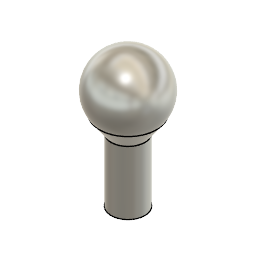
Ball Joint's Baseless Ball (Autodesk Fusion 360 design; units mm, degrees)
Autodesk Fusion 360 part; units mm, degrees
note: some values were not read from the file. Chosen so that the rebuilt part matches the saved one: which bodies a step acts on.
sphere "SpherePrimitive1" add diameter 12 placed x (1, 0, 0) y (0, 1, 0) z (0, 0, 1) at (0, 0, 0) makes body 1
sketch "Sketch2" plane through (0, 0, 0) normal (0, 0, 1) x (1, 0, 0)
  circle A0 centre (0, 0) radius 6
  line L0 (0, 0) -> (3, 0)
  line L1 (2.0741, 19.9496) -> (0, 19.9496)
  line L2 (0, 19.9496) -> (0, 0)
  line L3 (-3, 0) -> (-3, 17.2973)
  line L4 (-2.0741, 19.9496) -> (0, 19.9496)
  line L5 (0, 0) -> (-3, 0)
  line L6 (4.9203, 3.4337) -> (3, 6.1854)
  line L7 (-4.9203, 3.4337) -> (-3, 6.1854)
  line L8 (2.0741, 19.9496) -> (5.0741, 19.9496)
  line L9 (5.0741, 19.9496) -> (9.6681, 19.9496) construction
  line L10 (5.0741, 19.9496) -> (5.0741, 18.7496)
  line L11 (5.0741, 18.7496) -> (3, 17.2973)
  line L12 (-2.0741, 19.9496) -> (-5.0741, 19.9496)
  line L13 (-5.0741, 19.9496) -> (-5.0741, 18.7496)
  line L14 (-5.0741, 18.7496) -> (-3, 17.2973)
  line L15 (3, 0) -> (3, 5.1962)
  line L16 (3, 6.1854) -> (3, 17.2973)
  dimension "d2" = 3
  dimension "d4" = 3
  dimension "d6" = 1.2
  dimension "d7" = 125
  constraint horizontal L0
  constraint vertical L15
  constraint horizontal L1
  constraint vertical L2
  constraint coincident A0.centre L0.start
  constraint symmetric A0.centre L2 L0.start
  constraint symmetric L0.end L2 L3.start
  constraint symmetric L1.start L2 L4.start
  constraint symmetric L1.end L2 L4.end
  constraint coincident L6.end L15
  constraint tangent A0 L6
  constraint coincident A0 L6.start
  constraint symmetric L2 L6.end L7.end
  constraint symmetric L2 L6.start L7.start
  constraint perpendicular L8 L15
  constraint horizontal L9
  constraint perpendicular L9 L10
  constraint symmetric L2 L8.end L12.end
  constraint symmetric L2 L10.end L13.end
  constraint coincident A0 L15.end
  constraint collinear L15 L16
  measures "d2" distance of A0.centre L0.end
  measures "d4" distance of L1.start L8.end
  measures "d6" distance of L8.end L10.end
  measures "d7" angle of L10 L11
revolve "Revolve1" add sketch "Sketch2" angle 360 about axis through (0, 19.9496, 0) along (0, -1, 0) contours A0 L1 L2 L6 L8 L10 L11 L16 bodies 1
copy_body "Body->Comp1" bodies 1 removing the originals makes body 2 in component "ball"
sphere "SpherePrimitive2" add diameter 16 placed x (0, 0, -1) y (0, 1, 0) z (1, 0, 0) at (0, 0, 0) separate body makes body 3
sketch "Sketch4" plane through (0, 0, 0) normal (1, 0, 0) x (0, 0, -1)
  circle A0 centre (0, 0) radius 8
  line L0 (0, 0) -> (3, 0)
  line L1 (3, 0) -> (3, 20)
  line L2 (3, 20) -> (0, 20)
  line L3 (0, 20) -> (0, 0)
  line L4 (3, 20) -> (5, 20)
  line L5 (5, 20) -> (5, 18.5)
  line L6 (5, 18.5) -> (0, 14.999)
  line L7 (6.245, 5) -> (3, 9.053)
  dimension "d10" = 3
  dimension "d11" = 20
  dimension "d12" = 2
  dimension "d13" = 1.5
  dimension "d14" = 125
  dimension "d15" = 15
  constraint horizontal L0
  constraint vertical L1
  constraint horizontal L2
  constraint vertical L3
  constraint coincident A0.centre L0.start
  constraint perpendicular L1 L4
  constraint perpendicular L4 L5
  constraint coincident L3 L6.end
  constraint coincident A0 L7.start
  constraint coincident L1 L7.end
  constraint tangent A0 L7
  measures "d10" distance of A0.centre L0.end
  measures "d11" distance of A0.centre L2.end
  measures "d12" distance of L1.end L4.end
  measures "d13" distance of L4.end L5.end
  measures "d14" angle of L5 L6
  measures "d15" distance of L2 L7.start
revolve "Revolve2" add sketch "Sketch4" angle 360 about axis through (0, 20, 0) along (0, -1, 0) contours A0 L1 L7 | A0 L1 L3 L6 | L1 L2 L3 L6 | L1 L4 L5 L6 bodies 3
sphere "SpherePrimitive3" cut diameter 12 placed x (0, 0, -1) y (0, 1, 0) z (1, 0, 0) at (0, 0, 0) bodies 3
ref_plane "WorkPlane1" through (0, -3, 0) normal (0, 1, 0) x (0, 0, 1)
split "Split1" by plane through (0, -3, 0) normal (0, 1, 0) bodies 3 makes body 4 at (-1.7023, 1.8911, -7.5846)
chamfer "Chamfer1" distance 1 angle 60 1 edges at (-1.879, -3, 4.8445) measured on face at (-1.2767, 1.4183, -5.6884) on bodies 4
sketch "Sketch6" plane through (0, 0, 0) normal (1, 0, 0) x (0, 0, -1)
  line L0 (7.4162, -3) -> (-7.4162, -3) construction
  line L1 (-5, 20) -> (5, 20) construction
  line L2 (-5, 20) -> (-5, 18.5) construction
  line L3 (5, 20) -> (5, 18.5) construction
  line L4 (3, 17.0996) -> (5, 18.5) construction
  line L5 (-3, 17.0996) -> (-5, 18.5) construction
  line L6 (-3, 17.0996) -> (-3, 9.053) construction
  line L7 (3, 17.0996) -> (3, 9.053) construction
  line L8 (-3, 9.053) -> (-6.245, 5) construction
  line L9 (3, 9.053) -> (6.245, 5) construction
  arc A0 (-6.245, 5) -> (-7.4162, -3) centre (0, 0) ccw construction
  arc A1 (7.4162, -3) -> (6.245, 5) centre (0, 0) ccw construction
  line L10 (0, -3) -> (-1.5, -3)
  line L11 (-1.5, -3) -> (-1.5, 3)
  line L12 (0, 3) -> (0, -3)
  line L13 (1.5, -3) -> (1.5, 3)
  line L14 (0, -3) -> (1.5, -3)
  arc A2 (1.5, 3) -> (-1.5, 3) centre (0, 3) ccw
  dimension "d21" = 1.5
  dimension "d22" = 6
  constraint horizontal L10
  constraint vertical L11
  constraint vertical L12
  constraint midpoint L0 L10.start
  constraint coincident L12.start A2.centre
  constraint symmetric L10.start L12 L14.start
  constraint symmetric L10.end L12 L13.start
  constraint symmetric L11.end L12 L13.end
  measures "d21" distance of L10.start L10.end
  measures "d22" distance of L10.start L12.start
extrude "Extrude1" cut sketch "Sketch6" along normal mid plane 43 bodies 4
copy_body "CopyPasteBodies1" bodies 4 makes body 5
move_body "Move1" bodies 5 to x (1, 0, 0) y (0, 1, 0) z (0, 0, 1) at (0, 0, -20)
sketch "Sketch7" plane through (0, 0, 0) normal (0, 0, 1) x (1, 0, 0)
  line L0 (0, -3) -> (-1.5, -3)
  line L1 (-1.5, -3) -> (-1.5, 3)
  line L2 (7.2629, -3) -> (-7.2629, -3)
  line L3 (1.5, -3) -> (1.5, 3)
  line L4 (0, -3) -> (1.5, -3)
  arc A0 (1.5, 3) -> (-1.5, 3) centre (0, 3) ccw
  dimension "d25" = 1.5
  constraint horizontal L0
  constraint vertical L1
  constraint midpoint L0.start L2
  measures "d25" distance of L0.start L0.end
extrude "Extrude2" cut sketch "Sketch7" along normal mid plane 18 bodies 4
copy_body "Body->Comp2" bodies 5 removing the originals makes body 6 in component "Component"
copy_body "Body->Comp3" bodies 4 removing the originals makes body 7 in component "Component'"
move_body "Move1'" bodies 2 to x (1, 0, 0) y (0, -1, 0) z (0, 0, -1) at (0, 17, -9) in component "ball"
move_body "Move1''" bodies 7 to x (0.756992, 0, 0.653424) y (0, -1, 0) z (0.653424, 0, -0.756992) at (0, 17.106, 0) in component "Component'"
move_body "Move1'''" bodies 6 to x (1, 0, 0) y (0, -1, 0) z (0, 0, -1) at (0, 17.1992, -40) in component "Component"
extrude "Extrude1'" cut 1 faces at (-0.6782, -2.9496, -9.6705) along direction (0, 1, 0) blind 2.7 on bodies 2 bodies 2 in component "ball"
move_face "OffsetFaces1" offset -0.1 1 faces at (2.9851, 3.4385, -9.2987) on bodies 2 in component "ball"
component "ball" placed x (1, 0, 0) y (0, 1, 0) z (0, 0, 1) at (0, 0, 25)
hidden bodies 3
